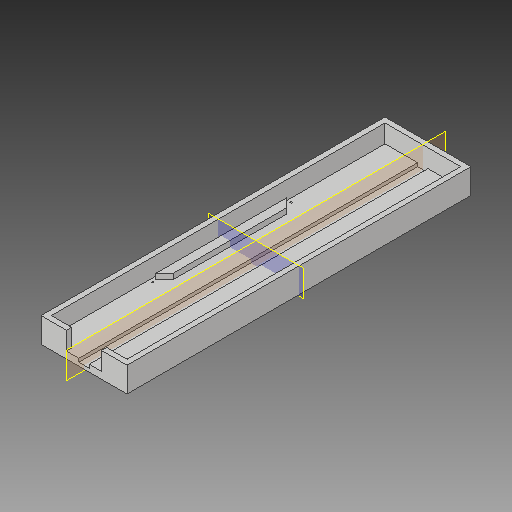
# Autodesk Inventor part: Base
Saved by Autodesk Inventor 2017 (Build 210142000, 142)
## iProperties
Created: 2017-01-18
Part Number: Base
Material: Generic
Document SubType Name: Modeling
Designer: A. Matías Quezada
Density: 1 g/cm^3
Appearance: Default
Author: A. Matías Quezada
Autodesk Inventor part; units mm, degrees
ref_plane "YZ Plane" through (0, 0, 0) normal (1, 0, 0) x (0, 1, 0)
ref_plane "XZ Plane" through (0, 0, 0) normal (0, 1, 0) x (-1, 0, 0)
ref_plane "XY Plane" through (0, 0, 0) normal (0, 0, 1) x (1, 0, 0)
sketch "Sketch1" plane through (0, 0, 0) normal (0, 1, 0) x (-1, 0, 0)
  line L0 (0, 0) -> (50, 0)
  line L1 (50, 0) -> (50, 200)
  line L2 (50, 200) -> (0, 200)
  line L3 (0, 200) -> (0, 0)
  dimension "d1" = 50
  dimension "d2" = 200
  constraints: 8 end point, 2 parallel, 1 horizontal, 1 perpendicular
  measures "d1" distance of L2.end L1.end
  measures "d2" distance of L1.end L0.end
extrude "Base" add sketch "Sketch1" along normal blind 4
sketch "Sketch3" plane through (0, 4, 0) normal (0, 1, 0) x (1, 0, 0)
  line L0 (-50, 0) -> (-50, -200) projected
  line L1 (-50, -200) -> (0, -200) projected
  line L2 (0, -200) -> (0, 0) projected
  line L3 (0, 0) -> (-50, 0) projected
  line L4 (-47, -197) -> (-47, -3)
  line L5 (-47, -3) -> (-3, -3)
  line L6 (-3, -3) -> (-3, -197)
  line L7 (-3, -197) -> (-47, -197)
  line L8 (-25, -198.6939) -> (-25, 11.8917)
  line L9 (-35.2, -200) -> (-14.8, -200)
  line L10 (-14.8, -200) -> (-14.8, -197)
  line L11 (-14.8, -197) -> (-35.2, -197)
  line L12 (-35.2, -197) -> (-35.2, -200)
  point P0 (-25, 0)
  point P1 (-25, -200)
  point P2 (-25, -197)
  dimension "d10" = 3
  dimension "d11" = 20.4
  constraints: 18 end point, 5 midpoint, 2 parallel, 1 horizontal, 1 perpendicular, 1 point on line, 1 vertical, 3 other
  measures "d10" distance between parallel lines of L0 L4
  measures "d11" distance between parallel lines of L10 L12
extrude "Muros" add sketch "Sketch3" along normal blind 10.5 contours L3 L8 L5 L4 L7 L12 L1 L0 | L3 L2 L1 L10 L7 L6 L5 L8
sketch "Sketch4" plane through (0, 4, 0) normal (0, 1, 0) x (1, 0, 0)
  line L0 (-35.2, -200) -> (-14.8, -200) projected
  line L1 (-47, -3) -> (-3, -3) projected
  line L2 (-28, -200) -> (-22, -200)
  line L3 (-22, -200) -> (-22, -3)
  line L4 (-22, -3) -> (-28, -3)
  line L5 (-28, -3) -> (-28, -200)
  line L6 (-3, -3) -> (-47, -3) projected
  point P0 (0, 0)
  point P1 (-25, -3)
  point P2 (-25, -3)
  point P3 (-25, -200)
  dimension "d14" = 6
  constraints: 8 end point, 5 midpoint, 2 parallel, 1 horizontal, 1 perpendicular
  measures "d14" distance between parallel lines of L3 L5
extrude "Rail" cut sketch "Sketch4" against normal blind 2
sketch "Sketch5" plane through (0, 4, 0) normal (0, 1, 0) x (1, 0, 0)
  line L0 (-45.2, -138) -> (-40.2, -138)
  line L1 (-40.2, -138) -> (-40.2, -62)
  line L2 (-40.2, -62) -> (-45.2, -62)
  line L3 (-45.2, -62) -> (-45.2, -138)
  line L4 (-9.8, -138) -> (-4.8, -138)
  line L5 (-4.8, -138) -> (-4.8, -62)
  line L6 (-4.8, -62) -> (-9.8, -62)
  line L7 (-9.8, -62) -> (-9.8, -138)
  line L8 (-28, -200) -> (-28, -3) projected
  line L9 (-22, -3) -> (-22, -200) projected
  line L10 (-35.2, -200) -> (-28, -200) projected
  line L11 (-22, -200) -> (-14.8, -200) projected
  line L12 (-40.2, -138) -> (-28, -138)
  line L13 (-9.8, -138) -> (-22, -138)
  line L14 (-22, -3) -> (-22, -200) projected
  line L15 (-40.2, -138) -> (-40.2, -200)
  point P0 (0, 0)
  dimension "d17" = 30.4
  dimension "d18" = 62
  dimension "d19" = 76
  dimension "d20" = 5
  constraints: 22 end point, 5 point on line, 4 parallel, 4 perpendicular, 3 equal length, 2 horizontal
  measures "d17" distance between parallel lines of L1 L7
  measures "d18" distance of L0.end L15.end
  measures "d19" distance of L2.end L0.start
  measures "d20" distance of L1.end L2.end
extrude "Extrusion4" add sketch "Sketch5" along normal blind 3.2
draft "FaceDraft1" angle 45 pull direction (1, 0, 0) faces at (-43.5333, 5.0667, 138) fixed edges at (-45.2, 5.6, 138)
draft "FaceDraft2" angle 45 pull direction (1, 0, 0) faces at (-41.8667, 5.0667, 62) fixed edges at (-45.2, 5.6, 62)
draft "FaceDraft3" angle 45 pull direction (-1, 0, 0) faces at (-8.1333, 5.0667, 138) fixed edges at (-4.8, 5.6, 138)
draft "FaceDraft4" angle 45 pull direction (-1, 0, 0) faces at (-6.4667, 5.0667, 62) fixed edges at (-4.8, 5.6, 62)
ref_plane "Work Plane1" through (0, 0, 100) normal (0, 0, -1) x (-1, 0, 0)
ref_plane "Work Plane2" through (-25, 0, 200) normal (1, 0, 0) x (0, 0, -1)
sketch "Sketch6" plane through (0, 4, 0) normal (0, 1, 0) x (1, 0, 0)
  line L0 (-45.2, -62) -> (-40.2, -67) projected
  line L1 (-45.2, -138) -> (-45.2, -62) projected
  line L2 (-47, -3) -> (-47, -197) projected
  line L3 (-40.2, -133) -> (-45.2, -138) projected
  point P0 (0, 0)
  point P1 (-44.8, -59.8)
  point P2 (-44.8, -140.2)
  dimension "d27" = 2.2
  dimension "d28" = 2.2
  dimension "d29" = 2.2
  dimension "d30" = 2.2
  measures "d27" distance from line of L2 point (-44.8, -59.8)
  measures "d28" vertical distance of L0.start point (-44.8, -59.8)
  measures "d29" distance from line of L2 point (-44.8, -140.2)
  measures "d30" vertical distance of L1.start point (-44.8, -140.2)
hole "Hole1" at (-44.8, 4, 59.8) at (-44.8, 4, 140.2) direction (0, -1, 0) diameter 1 end through all
equation "\"d1\" = base_ancho"
equation "\"d2\" = base_largo"
equation "\"d4\" = base_grosor"
equation "\"d10\" = base_muros_grosor"
equation "\"d11\" = base_muros_separación"
equation "\"d12\" = base_muros_alto"
equation "\"d14\" = base_rail_ancho"
equation "\"d15\" = base_rail_profundidad"
equation "\"d17\" = hoja_ancho + 2 * hoja_diente_ancho + 2 * general_margen"
equation "\"d18\" = -0.5 * base_deslizador_largo + 0.5 * base_largo"
equation "\"d19\" = base_deslizador_largo"
equation "\"d20\" = base_deslizador_ancho"
equation "\"d21\" = base_deslizador_alto"
equation "\"d23\" = base_deslizador_agarre"
equation "\"d24\" = base_deslizador_agarre"
equation "\"d25\" = base_deslizador_agarre"
equation "\"d26\" = base_deslizador_agarre"
equation "\"d27\" = base_traba_y"
equation "\"d28\" = base_traba_x"
equation "\"d29\" = base_traba_y"
equation "\"d30\" = base_traba_x"
equation "\"d31\" = traba_eje_diametro"
equation "\"base_ancho\" = 50"
equation "\"base_largo\" = 200"
equation "\"base_grosor\" = 4"
equation "\"base_muros_grosor\" = 3"
equation "\"base_muros_separación\" = 20.4"
equation "\"base_muros_alto\" = 10.5"
equation "\"base_rail_ancho\" = 6"
equation "\"base_rail_profundidad\" = 2"
equation "\"hoja_ancho\" = 20"
equation "\"hoja_diente_ancho\" = 5"
equation "\"general_margen\" = 0.2"
equation "\"base_deslizador_largo\" = 76"
equation "\"base_deslizador_ancho\" = 5"
equation "\"base_deslizador_alto\" = 3.2"
equation "\"base_deslizador_agarre\" = 45deg"
equation "\"traba_eje_diametro\" = 1"
equation "\"base_traba_y\" = 2.2"
equation "\"base_traba_x\" = 2.2"
body "Solid1"
